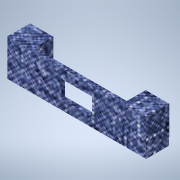
# Autodesk Inventor part: InternalSupportBracket
Saved by Autodesk Inventor 2020.1 (Build 241239000, 239)
## iProperties
Created: 2019-10-05
Part Number: InternalSupportBracket
Material: Generic
Document SubType Name: Modeling
Designer: Josiah
Density: 1 g/cm^3
Appearance: Denim - Blue
Author: Josiah
Autodesk Inventor part; units mm, degrees
ref_plane "YZ Plane" through (0, 0, 0) normal (1, 0, 0) x (0, 1, 0)
ref_plane "XZ Plane" through (0, 0, 0) normal (0, 1, 0) x (-1, 0, 0)
ref_plane "XY Plane" through (0, 0, 0) normal (0, 0, 1) x (1, 0, 0)
sketch "Sketch1" plane through (0, 0, 0) normal (0, 0, 1) x (1, 0, 0)
  line L0 (10.12, -21.6797) -> (-25.88, -21.6797)
  line L1 (-25.88, -21.6797) -> (-25.88, -12.1797)
  line L2 (-25.88, -12.1797) -> (10.12, -12.1797)
  line L3 (10.12, -12.1797) -> (10.12, -21.6797)
  line L4 (-3.88, -19.1797) -> (-11.88, -19.1797)
  line L5 (-11.88, -19.1797) -> (-11.88, -14.6797)
  line L6 (-11.88, -14.6797) -> (-3.88, -14.6797)
  line L7 (-3.88, -14.6797) -> (-3.88, -19.1797)
  line L8 (-20.9351, -12.1797) -> (-26.9351, -12.1797) construction
  point P0 (0, 0)
  point P1 (-7.88, -16.9297)
  dimension "d3" = 36
  dimension "d5" = 9.5
  dimension "d6" = 18
  dimension "d7" = 4.75
  dimension "d8" = 8
  dimension "d9" = 4.5
  dimension "d10" = 2.25
  dimension "d11" = 4
  constraints: 18 end point, 4 parallel, 2 horizontal, 2 perpendicular, 1 other
  measures "d3" distance of L0.start L0.end
  measures "d5" distance of L0.end L1.end
  measures "d6" distance from line of L1 point (-7.88, -16.93)
  measures "d7" distance from line of L0 point (-7.88, -16.93)
  measures "d8" distance of L5.end L6.end
  measures "d9" distance of L4.end L5.end
  measures "d10" distance from line of point (-7.88, -16.93) L6
  measures "d11" distance from line of L5 point (-7.88, -16.93)
extrude "SUPPORT TABLE" add sketch "Sketch1" along normal blind 1
sketch "Sketch2" plane through (0, 0, 0) normal (0, 0, -1) x (-1, 0, 0)
  line L0 (21.9351, -13.1797) -> (21.9351, -20.6797) construction
  line L1 (21.9351, -20.6797) -> (25.9351, -20.6797) construction
  line L2 (25.9351, -20.6797) -> (25.9351, -13.1797) construction
  line L3 (25.9351, -13.1576) -> (21.9351, -13.1576) construction
  line L4 (7.838, -23.7532) -> (7.838, -10.1502) construction
  line L5 (19.882, -21.6797) -> (19.882, -12.1797)
  line L6 (19.882, -12.1797) -> (25.882, -12.1797)
  line L7 (25.882, -12.1797) -> (25.882, -21.6797)
  line L8 (25.882, -21.6797) -> (19.882, -21.6797)
  line L9 (-5.118, -13.1797) -> (-5.118, -20.6797) construction
  line L10 (-5.118, -20.6797) -> (-9.118, -20.6797) construction
  line L11 (-9.118, -20.6797) -> (-9.118, -13.1797) construction
  line L12 (-9.118, -13.1797) -> (-5.118, -13.1797) construction
  line L13 (-4.12, -21.6797) -> (-4.12, -12.1797)
  line L14 (-4.12, -12.1797) -> (-10.12, -12.1797)
  line L15 (-10.12, -12.1797) -> (-10.12, -21.6797)
  line L16 (-10.12, -21.6797) -> (-4.12, -21.6797)
  line L17 (25.88, -21.6797) -> (25.88, -12.1797) construction
  line L18 (25.88, -12.1797) -> (-10.12, -12.1797) projected
  point P0 (0, 0)
  constraints: 26 end point, 1 horizontal alignment, 1 vertical
extrude "LEGS" add sketch "Sketch2" along normal blind 4.9
sketch "Sketch3" plane through (0, 0, 0) normal (0, 0, -1) x (-1, 0, 0)
  line L0 (25.882, -21.6797) -> (25.882, -12.1797) construction
  line L1 (19.882, -21.6797) -> (25.882, -21.6797) construction
  line L2 (19.882, -12.1797) -> (19.882, -21.6797) construction
  line L3 (19.882, -12.1797) -> (19.882, -21.6797) construction
  line L4 (19.882, -21.6797) -> (25.882, -21.6797) construction
  line L5 (25.882, -21.6797) -> (25.882, -12.1797) construction
  line L6 (25.882, -12.1797) -> (19.882, -12.1797) construction
  line L7 (-4.12, -12.1797) -> (-10.12, -12.1797) construction
  line L8 (-10.12, -12.1797) -> (-10.12, -21.6797) construction
  line L9 (-10.12, -21.6797) -> (-4.12, -21.6797) construction
  line L10 (-4.12, -21.6797) -> (-4.12, -12.1797) construction
  line L11 (24.882, -20.6797) -> (20.882, -20.6797)
  line L12 (20.882, -20.6797) -> (20.882, -13.1797)
  line L13 (20.882, -13.1797) -> (24.882, -13.1797)
  line L14 (24.882, -13.1797) -> (24.882, -20.6797)
  line L15 (7.838, -20.9409) -> (7.838, -12.9184) construction
  line L16 (-9.206, -20.6797) -> (-5.206, -20.6797)
  line L17 (-5.206, -20.6797) -> (-5.206, -13.1797)
  line L18 (-5.206, -13.1797) -> (-9.206, -13.1797)
  line L19 (-9.206, -13.1797) -> (-9.206, -20.6797)
  point P0 (0, 0)
  point P1 (7.838, -16.9297)
  point P2 (7.838, -16.9297)
  dimension "d24" = 1
  dimension "d25" = 1
  dimension "d26" = 1
  dimension "d27" = 1
  constraints: 18 end point, 4 symmetric about line, 2 parallel, 1 coincident, 1 horizontal, 1 midpoint, 1 perpendicular, 1 vertical, 1 other
  measures "d24" distance between parallel lines of L14 L0
  measures "d25" distance between parallel lines of L12 L2
  measures "d26" distance between parallel lines of L11 L1
  measures "d27" distance between parallel lines of L13 L6
extrude "PINS FOR LINEUP" add sketch "Sketch3" along normal blind 5.9
equation "\"d10\" = 0.5 * d9"
equation "\"d11\" = 0.5 * d8"
body "Solid1"
